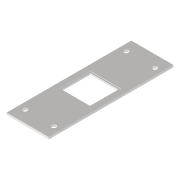
# Autodesk Inventor part: 40_microfluidic_chip_lightsheet_base_v0
Saved by Autodesk Inventor 2022 (Build 260153000, 153)
## iProperties
Created: 2021-12-21
Part Number: 40_microfluidic_chip_lightsheet_base_v0
Material: Generisch
Document SubType Name: Modeling
Designer: diederichbenedict
Density: 1 g/cm^3
Appearance: Vorgabe
Author: diederichbenedict
Autodesk Inventor part; units mm, degrees
ref_plane "YZ Plane" through (0, 0, 0) normal (1, 0, 0) x (0, 1, 0)
ref_plane "XZ Plane" through (0, 0, 0) normal (0, 1, 0) x (-1, 0, 0)
ref_plane "XY Plane" through (0, 0, 0) normal (0, 0, 1) x (1, 0, 0)
sketch "Skizze1" plane through (0, 0, 0) normal (0, 1, 0) x (-1, 0, 0)
  line L0 (12.5, -37) -> (-12.5, -37)
  line L1 (-12.5, -37) -> (-12.5, 37)
  line L2 (-12.5, 37) -> (12.5, 37)
  line L3 (12.5, 37) -> (12.5, -37)
  line L4 (12.5, -37) -> (-12.5, 37) construction
  line L5 (-12.5, -37) -> (12.5, 37) construction
  line L6 (8.5, 8.5) -> (-8.5, 8.5)
  line L7 (-8.5, 8.5) -> (-8.5, -8.5)
  line L8 (-8.5, -8.5) -> (8.5, -8.5)
  line L9 (8.5, -8.5) -> (8.5, 8.5)
  line L10 (8.5, 8.5) -> (-8.5, -8.5) construction
  line L11 (-8.5, 8.5) -> (8.5, -8.5) construction
  line L12 (-8.5, -30) -> (8.5, -30) construction
  line L13 (8.5, -30) -> (8.5, 30) construction
  line L14 (8.5, 30) -> (-8.5, 30) construction
  line L15 (-8.5, 30) -> (-8.5, -30) construction
  line L16 (-8.5, -30) -> (8.5, 30) construction
  line L17 (8.5, -30) -> (-8.5, 30) construction
  circle A0 centre (8.5, 30) radius 1.4
  circle A1 centre (-8.5, 30) radius 1.4
  circle A2 centre (8.5, -30) radius 1.4
  circle A3 centre (-8.5, -30) radius 1.4
  point P0 (0, 0)
  dimension "d0" = 25
  dimension "d1" = 74
  dimension "d2" = 17
  dimension "d3" = 17
  dimension "d10" = 17
  dimension "d11" = 60
  dimension "d12" = 2.8
  dimension "d13" = 2.8
  dimension "d14" = 2.8
  dimension "d15" = 2.8
  constraints: 36 end point, 6 midpoint, 6 parallel, 4 centre point, 4 coincident, 3 horizontal, 3 perpendicular
  measures "d0" distance of L1.end L2.end
  measures "d1" distance of L0.end L1.end
  measures "d2" distance of L8.end L7.end
  measures "d3" distance of L7.end L6.end
  measures "d10" distance of L14.end L13.end
  measures "d11" distance of L13.end L12.end
  measures "d12" diameter of A0
  measures "d13" diameter of A1
  measures "d14" diameter of A2
  measures "d15" diameter of A3
extrude "Extrusion1" add sketch "Skizze1" along normal blind 1
sketch "Skizze2" plane through (0, 1, 0) normal (0, 1, 0) x (1, 0, 0)
  line L0 (-12.5, -37) -> (12.5, -37) projected
  line L1 (12.5, -37) -> (12.5, 37) projected
  line L2 (12.5, 37) -> (-12.5, 37) projected
  line L3 (-12.5, 37) -> (-12.5, -37) projected
  line L4 (-8.5, -8.5) -> (-8.5, 8.5) projected
  line L5 (-8.5, 8.5) -> (8.5, 8.5) projected
  line L6 (8.5, 8.5) -> (8.5, -8.5) projected
  line L7 (8.5, -8.5) -> (-8.5, -8.5) projected
  line L8 (-9.25, -9.25) -> (9.25, -9.25)
  line L9 (9.25, -9.25) -> (9.25, 9.25)
  line L10 (9.25, 9.25) -> (-9.25, 9.25)
  line L11 (-9.25, 9.25) -> (-9.25, -9.25)
  line L12 (-9.25, -9.25) -> (9.25, 9.25) construction
  line L13 (9.25, -9.25) -> (-9.25, 9.25) construction
  circle A0 centre (-8.5, -30) radius 1.4 projected
  circle A1 centre (8.5, -30) radius 1.4 projected
  circle A2 centre (8.5, 30) radius 1.4 projected
  circle A3 centre (-8.5, 30) radius 1.4 projected
  point P0 (0, 0)
  dimension "d6" = 18.5
  dimension "d7" = 18.5
  constraints: 12 end point, 2 midpoint, 2 parallel, 1 horizontal, 1 perpendicular
  measures "d6" distance of L10.end L9.end
  measures "d7" distance of L9.end L8.end
extrude "Extrusion2" add sketch "Skizze2" along normal blind 0.3 contours L3 L2 L1 L0
